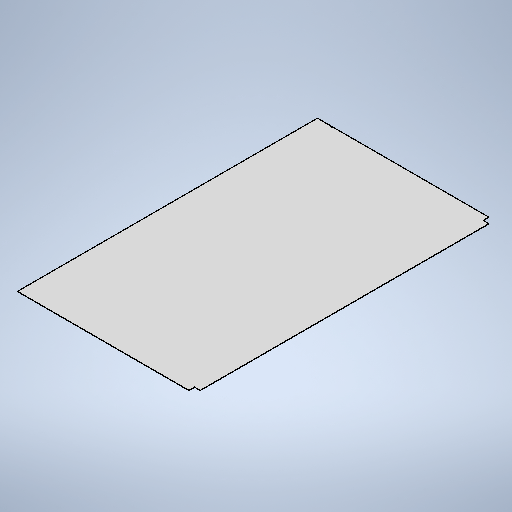
# Autodesk Inventor part: GnG frame 1.1 floor sheet
Saved by Autodesk Inventor 2025.3 (Build 293356000, 356)
## iProperties
Created: 2025-10-28
Part Number: GnG frame 1.1 floor sheet
Material: Stainless Steel
Document SubType Name: Sheet Metal
Designer: admin
Mass: 280.619 g
Surface Area: 364.406 cm^2
Volume: 35.0774 cm^3
Density: 8 g/cm^3
Sheet Metal Rule: AISI304 3mm Die 32
Sheet Metal Width: 1240,000 mm
Sheet Metal Length: 2100,000 mm
Sheet Metal Area: 2604000,000 mm^2
Appearance: Default
Stock Number: 1.1
Flat Pattern Width: 124 cm
Flat Pattern Length: 210 cm
Flat Pattern Area: 26040 cm^2
Author: admin
Autodesk Inventor part; units mm, degrees
ref_plane "YZ Plane" through (0, 0, 0) normal (1, 0, 0) x (0, 1, 0)
ref_plane "XZ Plane" through (0, 0, 0) normal (0, 1, 0) x (-1, 0, 0)
ref_plane "XY Plane" through (0, 0, 0) normal (0, 0, 1) x (1, 0, 0)
sketch "Sketch1" plane through (0, 0, 0) normal (0, 0, 1) x (1, 0, 0)
  line L0 (0, 0) -> (-1240, 0)
  line L1 (-1240, 0) -> (-1240, -2100)
  line L2 (-1240, -2100) -> (0, -2100)
  line L3 (0, -2100) -> (0, 0)
  line L4 (0, 0) -> (-40, 0)
  line L5 (-40, 0) -> (-40, -40)
  line L6 (-40, -40) -> (0, -40)
  line L7 (0, -40) -> (0, 0)
  line L8 (0, -2100) -> (-40, -2100)
  line L9 (-40, -2100) -> (-40, -2060)
  line L10 (-40, -2060) -> (0, -2060)
  line L11 (0, -2060) -> (0, -2100)
  point P0 (0, -40)
  point P1 (0, -2060)
  dimension "d22" = 1240
  dimension "d23" = 2100
  dimension "d24" = 40
  dimension "d25" = 40
  measures "d22" distance of L2.end L1.end
  measures "d23" distance of L1.end L0.end
  measures "d24" distance of L6.end L5.end
  measures "d25" distance of L5.end L4.end
extrude "Plate1" add sketch "Sketch1" along normal blind 3 contours L5 L6 L3 L10 L9 L2 L1 L0
sketch "Sketch5" plane through (0, 0, 3) normal (0, 0, 1) x (1, 0, 0)
  line L0 (-1240, -2100) -> (-1240, 0) projected
  line L1 (-40, -2100) -> (-1240, -2100) projected
  line L2 (-40, -2060) -> (-40, -2100) projected
  line L3 (0, -2060) -> (-40, -2060) projected
  line L4 (0, -40) -> (0, -2060) projected
  line L5 (-40, -40) -> (0, -40) projected
  line L6 (-40, 0) -> (-40, -40) projected
  line L7 (-1240, 0) -> (-40, 0) projected
  line L8 (-1140, 0) -> (-1138, 0)
  line L9 (-1138, 0) -> (-1138, -5)
  line L10 (-1138, -5) -> (-1140, -5)
  line L11 (-1140, -5) -> (-1140, 0)
  line L12 (-1132, 0) -> (-1130, 0)
  line L13 (-1130, 0) -> (-1130, -5)
  line L14 (-1130, -5) -> (-1132, -5)
  line L15 (-1132, -5) -> (-1132, 0)
  line L16 (-1136, 0) -> (-1134, 0)
  line L17 (-1134, 0) -> (-1134, -5)
  line L18 (-1134, -5) -> (-1136, -5)
  line L19 (-1136, -5) -> (-1136, 0)
  line L20 (-1240, 0) -> (-40, 0) projected
  line L21 (-1138, -2.5) -> (-1136, -2.5)
  line L22 (-1128, 0) -> (-1125, 0)
  line L23 (-1134, -2.5) -> (-1132, -2.5)
  line L24 (-1128, 0) -> (-1126.9884, -4.6072)
  arc A0 (-1126.9884, -4.6072) -> (-1126.0116, -4.6072) centre (-1126.5, -4.5) ccw
  line L25 (-1126.0116, -4.6072) -> (-1125, 0)
  line L26 (-1130, 0) -> (-1128, 0)
  line L27 (-1123, 0) -> (-1121, 0)
  line L28 (-1121, 0) -> (-1121, -5)
  line L29 (-1121, -5) -> (-1123, -5)
  line L30 (-1123, -5) -> (-1123, 0)
  line L31 (-1115, 0) -> (-1113, 0)
  line L32 (-1113, 0) -> (-1113, -5)
  line L33 (-1113, -5) -> (-1115, -5)
  line L34 (-1115, -5) -> (-1115, 0)
  line L35 (-1119, 0) -> (-1117, 0)
  line L36 (-1117, 0) -> (-1117, -5)
  line L37 (-1117, -5) -> (-1119, -5)
  line L38 (-1119, -5) -> (-1119, 0)
  line L39 (-1121, -2.5) -> (-1119, -2.5)
  line L40 (-1117, -2.5) -> (-1115, -2.5)
  line L41 (-1125, 0) -> (-1123, 0)
  line L42 (-40, 0) -> (-1240, 0) projected
  circle A1 centre (-1145, 0) radius 1.5
  point P0 (0, 0)
  point P1 (-1131, 0)
  point P2 (-1135, 0)
  point P3 (-1126.5, 0)
  point P4 (-1114, 0)
  point P5 (-1118, 0)
  point P6 (-1122, 0)
  point P7 (-1143.5, 0)
  point P8 (-1146.5, 0)
  dimension "d34" = 2
  dimension "d35" = 5
  dimension "d36" = 0.5
  dimension "d37" = 100
  dimension "d40" = 3
  dimension "d41" = 2
  dimension "d42" = 5
  dimension "d43" = 3
  dimension "d44" = 5
  constraints: 66 end point, 14 midpoint, 12 parallel, 10 equal length, 10 horizontal, 6 perpendicular, 4 collinear, 3 tangent, 2 centre point, 2 point on circle, 1 point on line, 1 vertical alignment, 8 other
  measures "d34" distance of L9.end L10.end
  measures "d35" distance of L10.end L8.start
  measures "d36" radius of A0
  measures "d37" distance between parallel lines of L0 L11
  measures "d40" distance of L22.start L22.end
  measures "d41" distance of L29.start L29.end
  measures "d42" distance of L29.end L27.start
  measures "d43" diameter of A1
  measures "d44" distance of A1.centre L8.start
extrude "Cut1" cut sketch "Sketch5" against normal blind 3 contours L7 A1 | L7 L9 L10 L11 picked at (-1145.0603, -0.4964)
equation "\"d25\" = d24"
equation "\"d36\" = 0.25 * d34"
equation "\"d38\" = Thickness"
equation "\"d2\" = Thickness"
equation "\"BendReliefWidth\" = Thickness"
equation "\"BendReliefDepth\" = 0.5 * Thickness"
equation "\"CornerReliefSize\" = 4 * Thickness"
equation "\"MinimumRemnant\" = 2 * Thickness"
equation "\"TransitionRadius\" = BendRadius"
equation "\"JacobiRadiusSize\" = BendRadius"
equation "\"GapSize\" = Thickness"
equation "\"Thickness\" = 3"
equation "\"BendRadius\" = 5"
body "Solid1"
